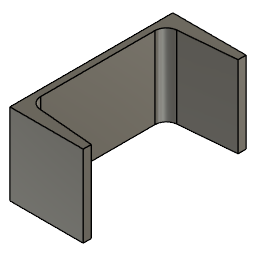
C-200×90×8×13.5 (Autodesk Fusion 360 design; units mm, degrees)
Autodesk Fusion 360 part; units mm, degrees
note: some values were not read from the file. Set by a fixed rule: which sketch regions a step uses.
sketch "スケッチ1" plane through (0, 0, 0) normal (0, 0, 1) x (1, 0, 0)
  arc A0 (20.7798, 184.0311) -> (8, 170.0843) centre (22, 170.0843) ccw
  line L0 (90, 190.087) -> (20.7798, 184.0311)
  line L1 (0, 200) -> (0, 0)
  line L2 (8, 170.0843) -> (8, 29.9157)
  line L3 (0, 0) -> (90, 0)
  line L4 (20.7798, 15.9689) -> (90, 9.913)
  arc A1 (8, 29.9157) -> (20.7798, 15.9689) centre (22, 29.9157) ccw
  line L5 (90, 9.913) -> (90, 0)
  line L6 (0, 200) -> (90, 200)
  line L7 (90, 200) -> (90, 190.087)
extrude "押し出し1" add sketch "スケッチ1" along normal blind 100
